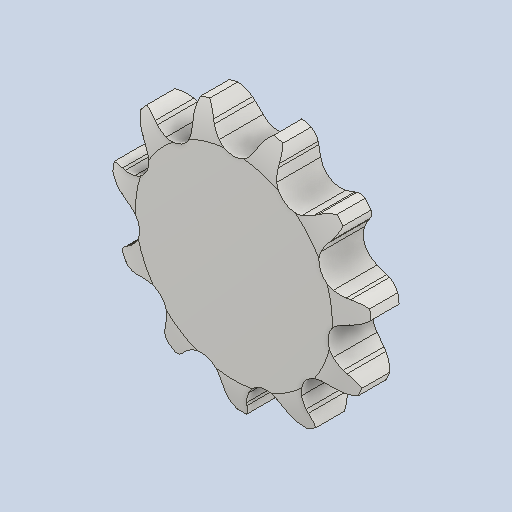
# Autodesk Inventor part: Rueda dentada de cadena de rodillos2
Saved by Autodesk Inventor 2022.1 (Build 261234000, 234)
## iProperties
Created: 2021-09-11
Part Number: Rueda dentada de cadena de rodillos2
Material: Steel
Document SubType Name: Modeling
Designer: seb_0
Density: 1 g/cm^3
Appearance: Steel
CustomPartVersion: 1
Author: seb_0
Autodesk Inventor part; units mm, degrees
ref_plane "YZ Plane" through (0, 0, 0) normal (1, 0, 0) x (0, 1, 0)
ref_plane "XZ Plane" through (0, 0, 0) normal (0, 1, 0) x (-1, 0, 0)
sketch "Perfil de diente teórico" plane through (0, 0, 0) normal (0, 0, 1) x (1, 0, 0)
  circle A0 centre (0, 0) radius 44.3683 construction
  line L0 (0, 0) -> (0, 44.3683) construction
  line L1 (0, 0) -> (23.9873, 37.325) construction
  circle A1 centre (0, 0) radius 50.0711
  arc A2 (-5.764, 39.4533) -> (5.764, 39.4533) centre (0, 44.3683) ccw
  line L2 (0, 44.3683) -> (23.9873, 37.325) construction
  line L3 (0, 44.3683) -> (9.1311, 52.1545) construction
  line L4 (9.1311, 52.1545) -> (-8.225, 43.102) construction
  arc A3 (12.3695, 48.5192) -> (8.8685, 44.3357) centre (20.1494, 38.4519) ccw
  arc A4 (-8.8685, 44.3357) -> (-12.3695, 48.5192) centre (-20.1494, 38.4519) ccw
  line L5 (-20.1494, 38.4519) -> (-8.8685, 44.3357) construction
  arc A5 (-8.225, 43.102) -> (-5.764, 39.4533) centre (9.1311, 52.1545) ccw
  line L6 (-8.225, 43.102) -> (-8.8685, 44.3357)
  arc A6 (5.764, 39.4533) -> (8.225, 43.102) centre (-9.1311, 52.1545) ccw
  line L7 (8.8685, 44.3357) -> (8.225, 43.102)
  line L8 (0, 0) -> (14.1067, 48.0429) construction
  point P0 (11.9937, 40.8467)
  dimension "d0" = 88.7366
  dimension "d2" = 32.727
  dimension "d3" = 7.575
  dimension "d10" = 130.455
  dimension "d11" = 12.909
  dimension "d12" = 12
  dimension "d13" = 19.575
  dimension "d14" = 21
  dimension "d23" = 7.5
  constraints: 18 end point, 15 point on circle, 7 centre point, 3 coincident, 3 point on line, 3 symmetric about line, 3 tangent, 1 equal radius, 1 midpoint, 1 parallel, 1 vertical, 1 other
  measures "d0" diameter of A0
  measures "d2" angle of L1 L0
  measures "d3" radius of A2
  measures "d10" angle of L3 L0
  measures "d11" angle of L4 L3
  measures "d12" distance of L2.start L3.end
  measures "d13" distance of L3.end L4.end
  measures "d14" distance of A3.centre L0.end
  measures "d23" distance from line of L8.end L2
sketch "Perfil de diente" plane through (0, 0, 0) normal (0, 0, 1) x (1, 0, 0)
  arc A0 (-6.9152, 41.2763) -> (6.9152, 41.2763) centre (0, 44.3683) ccw
  arc A1 (12.0626, 48.5964) -> (6.9152, 41.2763) centre (28.277, 31.7248) ccw
  arc A2 (-6.9152, 41.2763) -> (-12.0626, 48.5964) centre (-28.277, 31.7248) ccw
  line L0 (0, 0) -> (0, 44.3683) construction
  line L1 (0, 44.3683) -> (6.9152, 41.2763) construction
  line L2 (0, 44.3683) -> (-6.9152, 41.2763) construction
  circle A3 centre (0, 0) radius 50.0711 projected
  dimension "d44" = 131.818
  dimension "d45" = 23.4
  dimension "d46" = 7.575
  constraints: 9 point on circle, 6 end point, 3 centre point, 2 tangent, 1 coincident, 1 equal radius, 1 vertical, 1 other
  measures "d44" angle of L2 L1
  measures "d45" radius of A1
  measures "d46" radius of A0
sketch "Perfil de sección" plane through (0, 0, 0) normal (1, 0, 0) x (0, 1, 0)
  line L0 (50.0711, 0) -> (-50.0711, 0) projected
  line L1 (25.2911, 8.55) -> (-25.2911, 8.55)
  line L2 (-25.2911, 8.55) -> (-25.2911, -8.55)
  line L3 (-25.2911, -8.55) -> (25.2911, -8.55)
  line L4 (25.2911, -8.55) -> (25.2911, 8.55)
  line L5 (25.2911, 8.55) -> (50.0711, 8.55) construction
  line L6 (50.0711, 8.55) -> (50.0711, -8.55) construction
  line L7 (50.0711, -8.55) -> (25.2911, -8.55) construction
  line L8 (25.2911, -8.55) -> (25.2911, 8.55)
  arc A0 (50.0711, 5.425) -> (37.968, 8.55) centre (37.968, -16.45) ccw
  arc A1 (37.968, -8.55) -> (50.0711, -5.425) centre (37.968, 16.45) ccw
  line L9 (37.968, 8.55) -> (0, 8.55)
  line L10 (0, 8.55) -> (0, -8.55)
  line L11 (0, -8.55) -> (37.968, -8.55)
  line L12 (0, 8.55) -> (0, -8.55)
  line L13 (50.0711, 5.425) -> (50.0711, -5.425)
  point P0 (0, 0)
  point P1 (0, 0)
  dimension "d30" = 17.1
  dimension "d31" = 50.5822
  dimension "d32" = 17.1
  dimension "d33" = 3.125
  dimension "d34" = 25
  dimension "d43" = 8.55
  constraints: 26 end point, 7 midpoint, 5 perpendicular, 4 parallel, 4 point on circle, 3 point on line, 3 symmetric about line, 2 centre point, 2 horizontal, 2 tangent, 1 collinear, 1 other
  measures "d30" distance between parallel lines of L7 L5
  measures "d31" distance between parallel lines of L2 L4
  measures "d32" distance between parallel lines of L3 L1
  measures "d33" distance from line of L13.start L5
  measures "d34" radius of A0
  measures "d43" distance between parallel lines of L3 L0
revolve "Cubierta" add sketch "Perfil de sección" angle 360 about axis through (0, 0, 8.55) along (0, 0, -1) contours L10 L3 L2 L0 | L0 L2 L1 L10
revolve "Ramal" add sketch "Perfil de sección" angle 360 about axis through (0, 0, 8.55) along (0, 0, -1) contours L13 A1 L11 L4 L0 | L0 L4 L9 A0 L13 | L4 L3 L10 L0 | L0 L10 L1 L4
pattern_of_one "Patrón de ramal"
extrude "Diente teórico" cut sketch "Perfil de diente teórico" along normal through all both and the other way through all contours A3 L7 A6 A2 A5 L6 A4 A1 picked at (-0.3111, 45.5489)
extrude "Diente" [suppressed]
pattern_circular "Patrón de diente" count 11 over 360 about axis through (0, 0, -10) along (0, 0, 1) of "Diente teórico"
ref_plane "Plano síncrono" through (0, 44.3683, 0) normal (1, 0, 0) x (0, 1, 0)
equation "\"d3\" = 0.5 * da_Dr + da_SC"
equation "\"d12\" = 0.8 * da_Dr"
equation "\"d13\" = 1.3 * da_Dr + da_SC"
equation "\"d14\" = 1.4 * da_Dr"
equation "\"d23\" = da_Ha"
equation "\"d44\" = da_Alfa"
equation "\"d45\" = da_Re"
equation "\"d46\" = da_Ri"
equation "\"d30\" = da_Bf"
equation "\"d31\" = da_Ds"
equation "\"d32\" = da_Bs"
equation "\"d33\" = da_Ba"
equation "\"d34\" = da_Rx"
equation "\"d40\" = da_pt"
equation "\"form_type\" = 0"
equation "\"da_p\" = 25"
equation "\"da_Dr\" = 15"
equation "\"da_SC\" = 0.075"
equation "\"da_Ha\" = 7.5"
equation "\"da_pt\" = 32"
equation "\"da_Bf\" = 17.1"
equation "\"da_Ba\" = 3.125"
equation "\"da_Rx\" = 25"
equation "\"da_Ra\" = 1"
equation "\"da_Bs\" = 17.1"
equation "\"da_Ds\" = 50.58218"
equation "\"da_Re\" = 23.4"
equation "\"da_Ri\" = 7.575"
equation "\"da_Alfa\" = 131.818deg"
body "Solid1"
